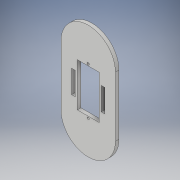
# Autodesk Inventor part: soporte servo base
Saved by Autodesk Inventor 2019 (Build 230136000, 136)
## iProperties
Created: 2020-02-10
Part Number: soporte servo base
Material: Generic
Document SubType Name: Modeling
Designer: jacqu
Density: 1 g/cm^3
Appearance: Default
base_servo: 20.000 mm
altura_servo: 40.000 mm
agujero_servo: 2.000 mm
distancia_agujero_servo: 1.750 mm
Author: jacqu
Autodesk Inventor part; units mm, degrees
ref_plane "YZ Plane" through (0, 0, 0) normal (1, 0, 0) x (0, 1, 0)
ref_plane "XZ Plane" through (0, 0, 0) normal (0, 1, 0) x (-1, 0, 0)
ref_plane "XY Plane" through (0, 0, 0) normal (0, 0, 1) x (1, 0, 0)
sketch "Sketch1" plane through (0, 0, 0) normal (0, 0, 1) x (1, 0, 0)
  line L0 (0, 0) -> (20, 0)
  line L1 (20, 0) -> (20, 40)
  line L2 (20, 40) -> (0, 40)
  line L3 (0, 40) -> (0, 0)
  line L4 (-15, -7.5) -> (-15, 47.5)
  line L5 (35, 47.5) -> (35, -7.5)
  arc A0 (35, 47.5) -> (-15, 47.5) centre (10, 47.5) ccw
  arc A1 (-15, -7.5) -> (35, -7.5) centre (10, -7.5) ccw
  dimension "base_servo" = 20
  dimension "altura_servo" = 40
  dimension "d2" = 15
  dimension "d3" = 15
  dimension "d4" = 55
  dimension "d5" = 55
  dimension "d9" = 7.5
  constraints: 12 end point, 4 point on circle, 3 tangent, 2 centre point, 2 parallel, 2 vertical, 1 horizontal, 1 perpendicular
  measures "base_servo" distance of L2.end L1.end
  measures "altura_servo" distance of L1.end L0.end
  measures "d2" distance between parallel lines of L4 L3
  measures "d3" distance between parallel lines of L5 L1
  measures "d4" distance of L4.start L4.end
  measures "d5" distance of L5.start L5.end
  measures "d9" distance from line of L0 A1.centre
extrude "Extrusion1" add sketch "Sketch1" along normal blind 3.3
sketch "Sketch2" plane through (0, 0, 3.3) normal (0, 0, 1) x (1, 0, 0)
  line L0 (22, 30.5) -> (25.3, 30.5)
  line L1 (25.3, 30.5) -> (25.3, 9.5)
  line L2 (25.3, 9.5) -> (22, 9.5)
  line L3 (22, 9.5) -> (22, 30.5)
  line L4 (-5.3, 30.5) -> (-2, 30.5)
  line L5 (-2, 30.5) -> (-2, 9.5)
  line L6 (-2, 9.5) -> (-5.3, 9.5)
  line L7 (-5.3, 9.5) -> (-5.3, 30.5)
  line L8 (0, 0) -> (0, 40) projected
  line L9 (20, 40) -> (20, 0) projected
  dimension "d12" = 3.3
  dimension "d13" = 3.3
  dimension "d14" = 21
  dimension "d16" = 9.5
  dimension "d17" = 2
  dimension "d18" = 2
  constraints: 16 end point, 4 parallel, 2 horizontal, 2 perpendicular, 2 point on line
  measures "d12" distance of L4.start L4.end
  measures "d13" distance of L0.start L0.end
  measures "d14" distance of L6.end L4.start
  measures "d16" distance from line of L8.end L4
  measures "d17" distance between parallel lines of L8 L5
  measures "d18" distance between parallel lines of L9 L3
extrude "Extrusion2" cut sketch "Sketch2" against normal blind 3.3
sketch "Sketch3" plane through (0, 0, 3.3) normal (0, 0, 1) x (1, 0, 0)
  circle A0 centre (10, 41.75) radius 1
  line L0 (0, 40) -> (20, 40) projected
  circle A1 centre (10, -1.75) radius 1
  line L1 (20, 0) -> (0, 0) projected
  dimension "agujero_servo" = 2
  dimension "distancia_agujero_servo" = 1.75
  dimension "d23" = 10
  dimension "d24" = 10
  dimension "d25" = 1.75
  constraints: 2 centre point, 1 equal radius
  measures "agujero_servo" diameter of A0
  measures "distancia_agujero_servo" distance from line of L0 A0.centre
  measures "d23" horizontal distance of A0.centre L1.end
  measures "d24" horizontal distance of L1.end A1.centre
  measures "d25" distance from line of L1 A1.centre
extrude "Extrusion3" cut sketch "Sketch3" against normal blind 3.3
equation "\"d3\" = d2"
equation "\"d5\" = d4"
equation "\"d9\" = 0.5 * d4 - 0.5 * altura_servo"
equation "\"d10\" = d12"
equation "\"d13\" = d12"
equation "\"d16\" = 0.5 * altura_servo - 0.5 * d14"
equation "\"d18\" = d17"
equation "\"d19\" = d12"
equation "\"d23\" = 0.5 * base_servo"
equation "\"d24\" = 0.5 * base_servo"
equation "\"d25\" = distancia_agujero_servo"
body "Solid1"
